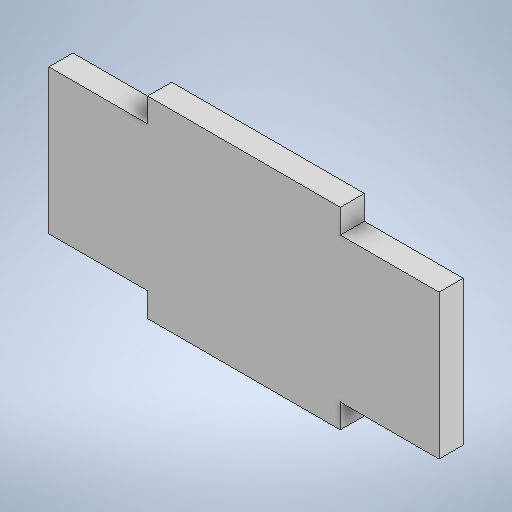
# Autodesk Inventor part: Path Base Fixation .2
Saved by Autodesk Inventor 2025.4 (Build 294407000, 407)
## iProperties
Created: 2026-04-10
Part Number: Path Base Fixation .2
Material: Generic
Document SubType Name: Sheet Metal
Designer: lenovo
Density: 1 g/cm^3
Sheet Metal Rule: Default_mm
Appearance: Default
Author: lenovo
Autodesk Inventor part; units mm, degrees
ref_plane "YZ Plane" through (0, 0, 0) normal (1, 0, 0) x (0, 1, 0)
ref_plane "XZ Plane" through (0, 0, 0) normal (0, 1, 0) x (-1, 0, 0)
ref_plane "XY Plane" through (0, 0, 0) normal (0, 0, 1) x (1, 0, 0)
sketch "Sketch1" plane through (0, 0, 0) normal (0, 0, 1) x (1, 0, 0)
  line L0 (-40.5, -15) -> (40.5, -15)
  line L1 (40.5, -15) -> (40.5, 15)
  line L2 (40.5, 15) -> (-40.5, 15)
  line L3 (-40.5, 15) -> (-40.5, -15)
  line L4 (-40.5, -15) -> (40.5, 15) construction
  line L5 (40.5, -15) -> (-40.5, 15) construction
  line L6 (-20, 20) -> (20, 20)
  line L7 (20, 20) -> (20, 15)
  line L8 (20, 15) -> (-20, 15)
  line L9 (-20, 15) -> (-20, 20)
  line L10 (-20, 20) -> (20, 15) construction
  line L11 (20, 20) -> (-20, 15) construction
  line L12 (-40.5, 0) -> (40.5, 0)
  line L13 (-20, -20) -> (20, -20)
  line L14 (20, -20) -> (20, -15)
  line L15 (20, -15) -> (-20, -15)
  line L16 (-20, -15) -> (-20, -20)
  line L17 (-20, -20) -> (20, -15) construction
  line L18 (20, -20) -> (-20, -15) construction
  point P0 (0, 0)
  point P1 (0, 17.5)
  point P2 (0, 15)
  point P3 (0, -17.5)
  point P4 (0, -15)
  dimension "d0" = 81
  dimension "d1" = 30
  dimension "d2" = 40
  dimension "d3" = 5
  measures "d0" distance of L2.end L1.end
  measures "d1" distance of L1.end L0.end
  measures "d2" distance of L6.start L6.end
  measures "d3" distance of L6.end L7.end
extrude "Plate1" add sketch "Sketch1" along normal blind 5
equation "\"d4\" = Thickness"
equation "\"BendRadius\" = Thickness"
equation "\"BendReliefWidth\" = Thickness"
equation "\"BendReliefDepth\" = 0.5 * Thickness"
equation "\"TransitionRadius\" = BendRadius"
equation "\"JacobiRadiusSize\" = BendRadius"
equation "\"GapSize\" = Thickness"
equation "\"Thickness\" = 5"
body "Solid1"
